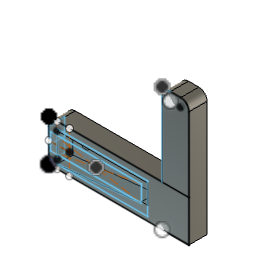
ServoArm v6 (Autodesk Fusion 360 design; units mm, degrees)
Autodesk Fusion 360 part; units mm, degrees
sketch "Sketch2" plane through (0, 0, 0) normal (0, 1, 0) x (1, 0, 0)
  line L0 (2, 0) -> (34, 0)
  line L1 (27.5, -10) -> (2, -10)
  line L2 (0, -8) -> (0, -2)
  line L3 (34, 0) -> (27.5, 0)
  arc A0 (0, -8) -> (2, -10) centre (2, -8) ccw
  arc A1 (2, 0) -> (0, -2) centre (2, -2) ccw
  line L4 (27.5, -10) -> (34, -10)
  line L5 (34, -10) -> (34, -28)
  line L6 (32, -30) -> (29.5, -30)
  line L7 (27.5, -28) -> (27.5, -10)
  arc A2 (27.5, -28) -> (29.5, -30) centre (29.5, -28) ccw
  arc A3 (32, -30) -> (34, -28) centre (32, -28) ccw
  line L8 (34, -10) -> (34, 0)
  line L9 (0, -5) -> (5, -5) construction
  point P0 (0, -10)
  point P1 (27.5, -30)
  dimension "d13" = 34
  dimension "d14" = 10
  dimension "d22" = 2
  dimension "d23" = 2
  dimension "d50" = 20
  dimension "d51" = 2
  dimension "d52" = 2
  dimension "d55" = 5
  constraint horizontal L0
  constraint horizontal L1
  constraint vertical L2
  constraint horizontal L3
  constraint coincident P0 L1
  constraint coincident P0 L2
  constraint tangent L1 A0
  constraint tangent L2 A0
  constraint coincident origin L0
  constraint coincident origin L2
  constraint tangent L0 A1
  constraint tangent L2 A1
  constraint horizontal L4
  constraint vertical L5
  constraint horizontal L6
  constraint vertical L7
  constraint coincident P1 L6
  constraint coincident P1 L7
  constraint tangent L6 A2
  constraint tangent L7 A2
  constraint tangent L5 A3
  constraint tangent L6 A3
  constraint perpendicular L3 L8
  constraint midpoint L2 L9.start
  constraint perpendicular L2 L9
  measures "d13" distance of origin L0.end
  measures "d14" distance of origin P0
  measures "d22" radius of A0
  measures "d23" radius of A1
  measures "d50" distance of L1.start P1
  measures "d51" radius of A2
  measures "d52" radius of A3
  measures "d55" distance of L9.start L9.end
extrude "Extrude1" add sketch "Sketch2" along normal blind 4.4 contours L0 L1 L2 L3 A0 A1 L4 L8
sketch "Sketch3" plane through (0, 0, 0) normal (0, 1, 0) x (1, 0, 0)
  line L0 (5, -10) -> (5, 0) construction
  line L1 (5, -5) -> (0, -5) construction
  line L2 (2, -10) -> (2, 0) construction
  line L3 (2, -8.488) -> (24, -8.488)
  line L4 (24, -8.488) -> (24, -0.988)
  line L5 (24, -0.988) -> (2, -0.988)
  line L6 (2, -0.988) -> (2, -8.488)
  line L7 (22.4627, -7.0337) -> (0.4627, -7.0337)
  line L8 (0.4627, -7.0337) -> (0.4627, -3.0337)
  line L9 (0.4627, -3.0337) -> (22.4627, -3.0337)
  line L10 (22.4627, -3.0337) -> (22.4627, -7.0337)
  line L11 (22.4627, -7.0337) -> (0.4627, -3.0337) construction
  line L12 (0.4627, -7.0337) -> (22.4627, -3.0337) construction
  line L13 (2, -0.988) -> (22.4627, -3.0337)
  point P0 (11.4627, -5.0337)
  dimension "d26" = 22
  dimension "d27" = 7.5
  dimension "d29" = 22
  dimension "d30" = 4
  constraint vertical L0
  constraint midpoint L0 L1.start
  constraint perpendicular L0 L1
  constraint horizontal L3
  constraint vertical L4
  constraint horizontal L5
  constraint vertical L6
  constraint coincident L2 L3.start
  constraint horizontal L7
  constraint perpendicular L7 L8
  constraint parallel L7 L9
  constraint parallel L8 L10
  constraint coincident L11 P0
  constraint coincident L12 P0
  measures "d26" distance of L3.start L3.end
  measures "d27" distance of L3.start L5.end
  measures "d29" distance of L8.end L9.end
  measures "d30" distance of L7.end L8.end
sketch "Sketch5" plane through (0, 0, 0) normal (1, 0, 0) x (0, 1, 0)
  line L0 (0, 8) -> (3.8, 8)
  line L1 (3.8, 8) -> (3.8, 0.5)
  line L2 (3.8, 0.5) -> (0, 0.5)
  line L3 (0, 0.5) -> (0, 8)
  line L4 (0, 8) -> (3.8, 8)
  line L5 (3.8, 8) -> (3.8, 4)
  line L6 (3.8, 4) -> (0, 4)
  line L7 (0, 4) -> (0, 8)
  dimension "d33" = 3.8
  dimension "d34" = 7.5
  dimension "d35" = 4
  constraint horizontal L0
  constraint vertical L1
  constraint horizontal L2
  constraint vertical L3
  constraint horizontal L4
  constraint vertical L5
  constraint horizontal L6
  constraint vertical L7
  measures "d33" distance of L0.start L0.end
  measures "d34" distance of L0.start L2.end
  measures "d35" distance of L0.start L6.end
extrude "Extrude2" cut sketch "Sketch5" along normal blind 22 from surface at 2 contours L0 L1 L3 L4 L5 L6 L7
extrude "Extrude3" cut sketch "Sketch3" along normal blind 3.8 contours L6 L7 L8 L9 | L6 L9 L13
extrude "Extrude4" cut sketch "Sketch3" along normal blind 3.8 contours L6 L7 L9 L10
extrude "Extrude5" add sketch "Sketch3" along normal blind 3.8 contours L6 L7 L8 L9
box "BoxPrimitive1" cut length 1.011 width 1.637 height 3.8 placed x (0, 0, -1) y (-1, 0, 0) z (0, 1, 0) at (23.991, 0, 4.3382)
extrude "Extrude6" add sketch "Sketch2" along normal blind 4.4 contours L4 L5 L6 L7 A2 A3
hole "Hole1" at (5.027, 4.4, 4.9908) direction (0, -1, 0) diameter 2.5 depth 2.5 tip angle 180
equation "machine_width = 81 mm"
equation "side_to_btn = 29 mm"
equation "box_width = 40 mm"
equation "holder_height = 11 mm"
equation "servo_height = 7.5 mm"
equation "servo_length = 22 mm"
equation "servo_depth = 3.8 mm"
equation "arm_base_length = 34 mm"
equation "arm_height = 10 mm"
equation "arm_depth = 4.4 mm"
equation "d13 = arm_base_length"
equation "d14 = arm_height"
equation "hook_length = 20 mm"
equation "hook_width = 6.5 mm"
equation "d24 = arm_depth"
equation "d26 = servo_length"
equation "d27 = servo_height"
equation "servo_height_end = 4 mm"
equation "d29 = servo_length"
equation "d30 = servo_height_end"
equation "d33 = servo_depth"
equation "d34 = servo_height"
equation "d35 = servo_height_end"
equation "d37 = servo_length"
equation "d39 = servo_depth"
equation "d41 = servo_depth"
equation "d43 = servo_depth"
equation "d47 = servo_depth"
equation "d53 = arm_depth"
